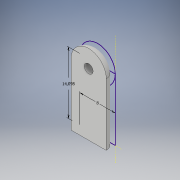
# Autodesk Inventor part: podpora
Saved by Autodesk Inventor 2019 (Build 230136000, 136)
## iProperties
Created: 2020-01-12
Part Number: podpora
Material: Ogólny
Document SubType Name: Modeling
Designer: Karolina
Density: 1 g/cm^3
Appearance: Domyślna
Author: Karolina
Autodesk Inventor part; units mm, degrees
ref_plane "YZ Plane" through (0, 0, 0) normal (1, 0, 0) x (0, 1, 0)
ref_plane "XZ Plane" through (0, 0, 0) normal (0, 1, 0) x (-1, 0, 0)
ref_plane "XY Plane" through (0, 0, 0) normal (0, 0, 1) x (1, 0, 0)
sketch "Szkic1" plane through (0, 0, 0) normal (0, 0, 1) x (1, 0, 0)
  line L0 (-9.6, 0) -> (1.6, 0) construction
  line L1 (0, -3.6196) -> (0, 21.7176) construction
  line L2 (0, 0) -> (-8, 0)
  line L3 (-8, 0) -> (-8, 14.098)
  line L4 (-8, 14.098) -> (0, 14.098)
  line L5 (0, 14.098) -> (0, 0)
  circle A0 centre (-4, 14.098) radius 4
  dimension "d1" = 8
  dimension "d2" = 14.098
  constraints: 8 end point, 2 parallel, 1 coincident, 1 horizontal, 1 horizontal alignment, 1 midpoint, 1 perpendicular, 2 other
  measures "d1" distance between parallel lines of L1 L3
  measures "d2" distance between parallel lines of L0 L4
extrude "Wyciągnięcie proste1" add sketch "Szkic1" along normal blind 2
hole "Otwór1" at (-4, 14.098, 0) direction (0, 0, 1) diameter 2 end through all
fillet "Zaokrąglenie1" radius 2 3 edges at (-4, 18.098, 0) (-8, 7.049, 0) (0, 7.049, 0)
